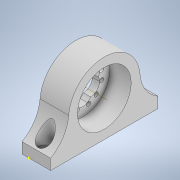
# Autodesk Inventor part: Motor Mount V2
Saved by Autodesk Inventor 2020 (Build 240168000, 168)
## iProperties
Created: 2020-01-13
Part Number: Motor Mount V2
Material: Generic
Document SubType Name: Modeling
Designer: maple
Density: 1 g/cm^3
Appearance: Default
Author: maple
Autodesk Inventor part; units mm, degrees
ref_plane "YZ Plane" through (0, 0, 0) normal (1, 0, 0) x (0, 1, 0)
ref_plane "XZ Plane" through (0, 0, 0) normal (0, 1, 0) x (-1, 0, 0)
ref_plane "XY Plane" through (0, 0, 0) normal (0, 0, 1) x (1, 0, 0)
sketch "Sketch1" plane through (0, 0, 0) normal (0, 1, 0) x (-1, 0, 0)
  line L0 (0, 0) -> (-20.32, 0)
  line L1 (-20.32, 0) -> (-20.32, -76.2)
  line L2 (-20.32, -76.2) -> (0, -76.2)
  line L3 (0, -76.2) -> (0, 0)
  dimension "d0" = 20.32
  dimension "d1" = 76.2
  constraints: 8 end point, 2 parallel, 1 horizontal, 1 perpendicular
  measures "d0" distance of L2.end L1.end
  measures "d1" distance of L1.end L0.end
extrude "Extrusion1" add sketch "Sketch1" along normal blind 7.62
sketch "Sketch2" plane through (0, 7.62, 0) normal (0, 1, 0) x (1, 0, 0)
  line L0 (0, 0) -> (0, 12.7)
  line L1 (0, 12.7) -> (20.32, 12.7)
  line L2 (20.32, 12.7) -> (20.32, 63.5)
  line L3 (20.32, 63.5) -> (0, 63.5)
  line L4 (0, 63.5) -> (0, 12.7)
  dimension "d4" = 12.7
  dimension "d5" = 20.32
  dimension "d6" = 50.8
  constraints: 10 end point, 2 parallel, 1 horizontal, 1 perpendicular, 1 vertical
  measures "d4" distance of L0.start L0.end
  measures "d5" distance of L3.end L2.end
  measures "d6" distance of L2.end L1.end
extrude "Extrusion2" add sketch "Sketch2" along normal blind 43.18
sketch "Sketch3" plane through (20.32, 0, 0) normal (1, 0, 0) x (0, 0, -1)
  line L0 (12.7, 50.8) -> (63.5, 50.8) projected
  line L1 (38.1, 50.8) -> (38.1, 25.4)
  circle A0 centre (38.1, 25.4) radius 19.05
  point P0 (0, 0)
  dimension "d9" = 25.4
  dimension "d10" = 38.1
  constraints: 2 end point, 1 centre point, 1 coincident, 1 midpoint, 1 vertical
  measures "d9" distance of L1.start L1.end
  measures "d10" diameter of A0
extrude "Extrusion3" cut sketch "Sketch3" against normal blind 15.24
sketch "Sketch4" plane through (5.08, 25.4, -38.1) normal (1, 0, 0) x (0, 0, -1)
  line L0 (0, 0) -> (0, 6.35)
  circle A0 centre (0, 6.35) radius 6.35
  point P0 (-38.1, -25.4)
  dimension "d13" = 6.35
  constraints: 2 end point, 1 coincident, 1 vertical, 1 vertical alignment, 2 other
  measures "d13" distance of L0.start L0.end
extrude "Extrusion4" cut sketch "Sketch4" against normal blind 15.24
sketch "Sketch5" plane through (5.08, 25.4, -38.1) normal (1, 0, 0) x (0, 0, -1)
  circle A0 centre (0, 6.35) radius 6.35 projected
  point P0 (-38.1, -25.4)
  point P1 (0, 0)
  constraints: 1 vertical alignment, 1 other
pattern_circular "Circular Pattern1" count 6 over 360 about axis through (5.08, 25.4, -38.1) along (1, 0, 0) of "Extrusion4"
fillet "Fillet1" radius 25.4 2 edges at (10.16, 50.8, -63.5) (10.16, 50.8, -12.7)
sketch "Sketch6" plane through (0, 7.62, 0) normal (0, 1, 0) x (1, 0, 0)
  line L0 (0, 0) -> (20.32, 0) projected
  line L1 (10.16, 0) -> (10.16, 6.35)
  line L2 (20.32, 76.2) -> (0, 76.2) projected
  line L3 (10.16, 76.2) -> (10.16, 69.85)
  dimension "d20" = 6.35
  dimension "d21" = 6.35
  constraints: 4 end point, 2 midpoint, 2 vertical
  measures "d20" distance of L1.start L1.end
  measures "d21" distance of L3.start L3.end
fillet "Fillet2" radius 25.4 2 edges at (10.16, 7.62, -63.5) (10.16, 7.62, -12.7)
hole "Hole1" at (10.16, 7.62, -6.35) at (10.16, 7.62, -69.85) direction (0, -1, 0) diameter 5.08 end through all counterbore diameter 10.16 counterbore depth 3.81
sketch "Sketch7" plane through (10.16, 7.62, -6.35) normal (0, -1, 0) x (1, 0, 0)
  circle A0 centre (0, 0) radius 5.08
  circle A1 centre (0, -63.5) radius 2.54 projected
  line L0 (-2.54, -63.5) -> (0, -63.5)
  circle A2 centre (0, -63.5) radius 5.08
  point P0 (-10.16, 6.35)
  dimension "d30" = 10.16
  dimension "d31" = 10.16
  constraints: 2 centre point, 2 end point, 1 coincident, 1 horizontal, 1 horizontal alignment, 1 other
  measures "d30" diameter of A0
  measures "d31" diameter of A2
extrude "Extrusion5" cut sketch "Sketch7" against normal blind 15.24 contours A0 | A1 | A2
sketch "Sketch8" plane through (0, 0, -76.2) normal (-1, 0, 0) x (0, 0, 1)
  arc A0 (32.6007, 15.875) -> (43.5993, 15.875) centre (38.1, 19.05) ccw projected
  line L0 (32.6007, 15.875) -> (43.5993, 34.925)
  arc A1 (43.5993, 34.925) -> (32.6007, 34.925) centre (38.1, 31.75) ccw projected
  line L1 (38.1, 31.75) -> (46.0552, 31.75) construction
  line L2 (41.275, 37.2493) -> (42.037, 38.5691)
  line L3 (38.1, 31.75) -> (44.45, 31.75) construction
  line L4 (34.925, 37.2493) -> (34.163, 38.5691)
  circle A2 centre (42.037, 38.5691) radius 1.524
  circle A3 centre (34.163, 38.5691) radius 1.524
  point P0 (76.2, 0)
  dimension "d35" = 1.524
  dimension "d37" = 1.524
  constraints: 10 end point, 2 coincident, 2 horizontal, 2 point on circle, 1 centre point, 1 tangent, 3 other
  measures "d35" distance of L2.start L2.end
  measures "d37" distance of L4.start L4.end
extrude "Extrusion6" cut sketch "Sketch8" against normal blind 15.24
pattern_circular "Circular Pattern2" count 6 over 360 about axis through (5.08, 25.4, -38.1) along (1, 0, 0) of "Extrusion6"
body "Solid1"
